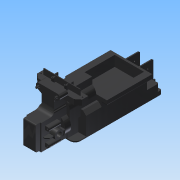
# Autodesk Inventor part: RearHousing
Saved by Autodesk Inventor 2014 (Build 180170000, 170)
## iProperties
Created: 2014-01-01
Part Number: RearHousing
Material: ABS Plastic
Document SubType Name: Modeling
Designer: davidgitz
Density: 1.06 g/cm^3
Appearance: Dark Gray
Author: davidgitz
Autodesk Inventor part; units mm, degrees
ref_plane "YZ Plane" through (0, 0, 0) normal (1, 0, 0) x (0, 1, 0)
ref_plane "XZ Plane" through (0, 0, 0) normal (0, 1, 0) x (-1, 0, 0)
ref_plane "XY Plane" through (0, 0, 0) normal (0, 0, 1) x (1, 0, 0)
sketch "Sketch1" plane through (0, 0, 0) normal (1, 0, 0) x (0, 1, 0)
  line L0 (28.5466, -43.7395) -> (-41.0494, -43.7395)
  line L1 (-41.0494, -43.7395) -> (-41.0494, 18.4905)
  line L2 (-41.0494, 18.4905) -> (-38.2554, 18.4905)
  line L3 (-38.2554, 18.4905) -> (-38.2554, 29.6665)
  line L4 (-38.2554, 29.6665) -> (20.9266, 29.6665)
  line L5 (20.9266, 29.6665) -> (20.9266, -2.0835)
  line L6 (28.5466, -43.7395) -> (28.5466, -14.2156)
  line L7 (33.9908, -15.5455) -> (15.8112, -15.5455) construction
  arc A0 (20.9266, -2.0835) -> (28.5466, -14.2156) centre (34.3947, -2.0835) ccw
  dimension "d13" = 62.23
  dimension "d15" = 2.794
  dimension "d16" = 11.176
  dimension "d17" = 59.182
  dimension "d18" = 31.75
  dimension "d19" = 28.194
  dimension "d20" = 7.62
  dimension "d21" = 69.596
  constraints: 16 end point, 5 parallel, 2 perpendicular, 2 point on circle, 1 centre point, 1 horizontal, 1 tangent
  measures "d13" distance of L0.end L1.end
  measures "d15" distance of L1.end L2.end
  measures "d16" distance of L2.end L3.end
  measures "d17" distance of L3.end L4.end
  measures "d18" distance of L4.end L5.end
  measures "d19" distance between parallel lines of L0 L7
  measures "d20" distance between parallel lines of L5 L6
  measures "d21" distance of L0.start L0.end
extrude "Extrusion1" add sketch "Sketch1" along normal mid plane 29.972
sketch "Sketch2" plane through (14.986, 0, 0) normal (1, 0, 0) x (0, 0, -1)
  line L0 (43.7395, -41.0494) -> (43.7395, 28.5466) projected
  line L1 (43.7395, 28.5466) -> (14.2156, 28.5466) projected
  arc A0 (2.0835, 20.9266) -> (14.2156, 28.5466) centre (2.0835, 34.3947) ccw projected
  line L2 (2.0835, 20.9266) -> (-29.6665, 20.9266) projected
  line L3 (-18.4905, -41.0494) -> (43.7395, -41.0494) projected
  line L4 (-18.4905, -41.0494) -> (-18.4905, 20.9266)
  point P0 (0, 0)
  constraints: 2 end point, 1 perpendicular, 1 point on line
extrude "Extrusion2" add sketch "Sketch2" along normal blind 2.54
mirror "Mirror1" about plane through (0, 0, 0) normal (1, 0, 0) of "Extrusion2"
fillet "Fillet1" radius 3.175 2 edges at (0, 20.9266, 29.6665) (0, -38.2554, 29.6665)
sketch "Sketch3" plane through (17.526, 0, 0) normal (1, 0, 0) x (0, 0, -1)
  line L0 (43.7395, -41.0494) -> (43.7395, 28.5466) projected
  line L1 (-18.4905, -41.0494) -> (43.7395, -41.0494) projected
  circle A0 centre (11.7355, -11.941) radius 10.414
  line L2 (0.9775, -22.355) -> (22.9537, -22.355) construction
  line L3 (22.1495, -2.7453) -> (22.1495, -21.5379) construction
  circle A1 centre (11.7355, -11.941) radius 6.096
  point P0 (0, 0)
  dimension "d27" = 20.828
  dimension "d28" = 18.6944
  dimension "d29" = 21.59
  dimension "d30" = 12.192
  constraints: 4 end point, 2 centre point, 2 tangent, 1 coincident, 1 parallel, 1 vertical
  measures "d27" diameter of A0
  measures "d28" distance between parallel lines of L1 L2
  measures "d29" distance between parallel lines of L0 L3
  measures "d30" diameter of A1
extrude "Extrusion3" add sketch "Sketch3" along normal blind 13.8684
sketch "Sketch4" plane through (17.526, -41.0494, -43.7395) normal (0, 0, -1) x (-1, 0, 0)
  arc A0 (0, 49.657) -> (0, 8.5598) centre (13.869, 29.1084) ccw
  line L0 (0, 49.657) -> (0, 8.5598)
  line L1 (-10.922, 46.5871) -> (-10.922, 14.6096) construction
  line L2 (0, 0) -> (35.052, 0) projected
  line L3 (0, 29.1084) -> (-28.8922, 29.1084) construction
  line L4 (0, 0) -> (0, 69.596) construction
  line L5 (0, 69.596) -> (0, 61.976) construction
  line L6 (0, 61.976) -> (0, 0) construction
  line L7 (0, 18.6944) -> (0, 39.5224) construction
  point P0 (17.526, 41.0494)
  dimension "d33" = 8.5598
  dimension "d39" = 29.1084
  dimension "d40" = 10.922
  constraints: 6 end point, 2 point on circle, 2 point on line, 1 centre point, 1 midpoint, 1 parallel, 1 perpendicular, 1 tangent
  measures "d33" distance of L2.start L0.end
  measures "d39" distance from line of L2 L3.start
  measures "d40" distance between parallel lines of L7 L1
extrude "Extrusion4" add sketch "Sketch4" against normal blind 13.97
sketch "Sketch5" plane through (17.526, 0, 0) normal (1, 0, 0) x (0, 0, -1)
  circle A0 centre (11.7355, -11.941) radius 10.414 projected
  line L0 (29.7695, -32.4896) -> (29.7695, 8.6076) projected
  line L1 (-18.4905, 20.9266) -> (-18.4905, -41.0494) projected
  line L2 (-8.7369, 10.284) -> (20.2191, 10.284)
  line L3 (20.2191, 10.284) -> (20.2191, 1.267)
  line L4 (20.2191, 1.267) -> (-8.7369, 1.267)
  line L5 (-8.7369, 1.267) -> (-8.7369, 10.284)
  line L6 (-8.2035, -11.941) -> (34.9388, -11.941) construction
  line L7 (-13.9185, -11.941) -> (-13.9185, -10.925)
  line L8 (-13.9185, -10.925) -> (1.3712, -10.925)
  line L9 (22.0998, -10.925) -> (29.7695, -10.925)
  line L10 (-5.7611, -1.527) -> (23.7536, -1.527) construction
  line L11 (-8.7369, -34.166) -> (20.2191, -34.166)
  line L12 (20.2191, -34.166) -> (20.2191, -25.149)
  line L13 (20.2191, -25.149) -> (-8.7369, -25.149)
  line L14 (-8.7369, -25.149) -> (-8.7369, -34.166)
  line L15 (-13.9185, -11.941) -> (-13.9185, -12.957)
  line L16 (-13.9185, -12.957) -> (1.3712, -12.957)
  line L17 (22.0998, -12.957) -> (29.7695, -12.957)
  arc A1 (1.3712, -10.925) -> (1.3712, -12.957) centre (11.7355, -11.941) ccw
  arc A2 (22.0998, -12.957) -> (22.0998, -10.925) centre (11.7355, -11.941) ccw
  line L18 (29.7695, -10.925) -> (29.7695, -12.957)
  point P0 (0, 0)
  point P1 (29.7695, -11.941)
  dimension "d41" = 28.956
  dimension "d42" = 9.017
  dimension "d43" = 9.7536
  dimension "d44" = 2.794
  dimension "d45" = 2.032
  dimension "d46" = 15.24
  constraints: 34 end point, 8 symmetric about line, 6 point on circle, 5 perpendicular, 4 point on line, 3 parallel, 2 centre point, 2 collinear, 1 coincident, 1 horizontal, 1 midpoint, 1 tangent
  measures "d41" distance of L2.start L2.end
  measures "d42" distance between parallel lines of L4 L2
  measures "d43" distance between parallel lines of L5 L1
  measures "d44" distance between parallel lines of L10 L4
  measures "d45" distance between parallel lines of L8 L16
  measures "d46" distance edge to line of A0 L7
extrude "Extrusion5" add sketch "Sketch5" along normal blind 10.16 contours A0 L9 L0 L17 | A0 L16 L15 L7 L8 | L2 L3 L4 L5 | L14 L13 L12 L11
chamfer "Chamfer1" distance 6.35 angle 45 1 edges at (27.686, -11.941, 13.9185)
sketch "Sketch6" plane through (17.526, 1.267, 8.7369) normal (0, 0, 1) x (1, 0, 0)
  line L0 (0, 0) -> (10.16, 0) projected
  circle A0 centre (5.6515, 4.5085) radius 1.5875
  arc A1 (10.16, 4.5085) -> (5.6515, 9.017) centre (5.6515, 4.5085) ccw
  line L1 (5.6515, 9.017) -> (10.16, 9.017)
  line L2 (10.16, 9.017) -> (10.16, 4.5085)
  line L3 (5.6515, 4.5085) -> (8.0267, 4.5085) construction
  arc A2 (5.6515, 0) -> (10.16, 4.5085) centre (5.6515, 4.5085) ccw
  line L4 (5.6515, 0) -> (10.16, 0)
  line L5 (10.16, 0) -> (10.16, 4.5085)
  point P0 (-17.526, -1.267)
  dimension "d52" = 3.175
  constraints: 10 end point, 4 point on circle, 3 centre point, 3 symmetric about line, 2 point on line, 1 coincident, 1 perpendicular, 1 tangent, 1 other
  measures "d52" diameter of A0
extrude "Extrusion6" cut sketch "Sketch6" against normal up to next
ref_plane "Work Plane1" through (17.526, -11.941, -11.7355) normal (0, 1, 0) x (1, 0, 0)
mirror "Mirror2" about plane through (17.526, -11.941, -11.7355) normal (0, 1, 0) of "Extrusion6"
mirror "Mirror3" about plane through (0, 0, 0) normal (1, 0, 0) of "Extrusion3", "Extrusion4", "Extrusion5", "Chamfer1", "Extrusion6", "Mirror2"
sketch "Sketch7" plane through (0, 0, 0) normal (1, 0, 0) x (0, 1, 0)
  arc A0 (28.5466, -14.2156) -> (34.3947, -15.5515) centre (34.3947, -2.0835) ccw
  arc A1 (20.9266, -2.0835) -> (28.5466, -14.2156) centre (34.3947, -2.0835) ccw projected
  line L0 (28.5466, -43.7395) -> (28.5466, -14.2156) projected
  line L1 (8.6076, -43.7395) -> (28.5466, -43.7395) projected
  line L2 (28.5466, -14.2156) -> (28.5466, -43.7395)
  line L3 (28.5466, -43.7395) -> (38.1986, -43.7395)
  line L4 (38.1986, -43.7395) -> (38.1986, -108.7635)
  line L5 (38.1986, -108.7635) -> (54.4546, -108.7635)
  line L6 (54.4546, -108.7635) -> (54.4546, -58.9795)
  line L7 (54.4546, -58.9795) -> (58.2646, -58.9795)
  line L8 (58.2646, -58.9795) -> (58.2646, -15.5515)
  line L9 (58.2646, -15.5515) -> (34.3947, -15.5515)
  line L10 (54.1292, -15.5515) -> (12.3088, -15.5515) construction
  point P0 (0, 0)
  dimension "d57" = 9.652
  dimension "d58" = 65.024
  dimension "d59" = 16.256
  dimension "d60" = 49.784
  dimension "d61" = 3.81
  dimension "d62" = 43.4279
  dimension "d63" = 29.718
  constraints: 18 end point, 5 parallel, 3 collinear, 2 concentric, 2 perpendicular, 2 point on circle, 1 centre point, 1 point on line, 1 tangent
  measures "d57" distance of L0.start L3.end
  measures "d58" distance of L3.end L4.end
  measures "d59" distance of L4.end L5.end
  measures "d60" distance of L5.end L6.end
  measures "d61" distance of L6.end L7.end
  measures "d62" distance of L7.end L8.end
  measures "d63" distance between parallel lines of L2 L8
extrude "Extrusion7" add sketch "Sketch7" along normal mid plane 29.972
fillet "Fillet2" radius 3.175 2 edges at (17.526, 28.5466, -28.9775) (-17.526, 28.5466, -28.9775)
fillet "Fillet3" radius 3.175 2 edges at (-14.986, 28.5466, -28.9775) (14.986, 28.5466, -28.9775)
sketch "Sketch9" plane through (-14.986, 34.3947, -15.5515) normal (0, 0, 1) x (1, 0, 0)
  line L0 (29.972, 23.8699) -> (29.972, 0) projected
  line L1 (0, 23.8699) -> (29.972, 23.8699) projected
  line L2 (0, 23.8699) -> (29.972, 23.8699)
  line L3 (29.972, 23.8699) -> (29.972, 11.4239)
  line L4 (29.972, 11.4239) -> (0, 11.4239)
  line L5 (0, 11.4239) -> (0, 23.8699)
  point P0 (14.986, -34.3947)
  dimension "d69" = 12.446
  constraints: 8 end point, 2 parallel, 1 horizontal, 1 perpendicular, 1 point on line
  measures "d69" distance between parallel lines of L1 L4
extrude "Extrusion8" cut sketch "Sketch9" against normal blind 19.558
sketch "Sketch10" plane through (-14.986, 34.3947, -35.1095) normal (0, 0, 1) x (1, 0, 0)
  line L0 (29.972, 23.8699) -> (29.972, 11.4239) projected
  line L1 (29.972, 11.4239) -> (0, 11.4239) projected
  line L2 (29.972, 11.4239) -> (29.972, 13.8369)
  line L3 (31.6529, 16.6384) -> (40.8193, 21.5272)
  line L4 (42.7792, 32.0645) -> (41.5897, 33.4399)
  line L5 (39.1882, 34.5379) -> (14.986, 34.5379)
  line L6 (14.986, 34.5379) -> (14.986, 11.4239) construction
  arc A0 (40.8193, 21.5272) -> (42.7792, 32.0645) centre (37.592, 27.5783) ccw
  line L7 (44.45, 35.5945) -> (44.45, 20.8192) construction
  arc A1 (41.5897, 33.4399) -> (39.1882, 34.5379) centre (39.1882, 31.3629) ccw
  arc A2 (31.6529, 16.6384) -> (29.972, 13.8369) centre (33.147, 13.8369) ccw
  line L8 (0, 13.8369) -> (0, 11.4239)
  line L9 (0, 11.4239) -> (0, 13.8369)
  line L10 (-1.6809, 16.6384) -> (-10.8473, 21.5272)
  line L11 (-12.8072, 32.0645) -> (-11.6177, 33.4399)
  line L12 (-9.2162, 34.5379) -> (14.986, 34.5379)
  arc A3 (-12.8072, 32.0645) -> (-10.8473, 21.5272) centre (-7.62, 27.5783) ccw
  line L13 (-14.478, 35.5945) -> (-14.478, 20.8192) construction
  arc A4 (-9.2162, 34.5379) -> (-11.6177, 33.4399) centre (-9.2162, 31.3629) ccw
  arc A5 (0, 13.8369) -> (-1.6809, 16.6384) centre (-3.175, 13.8369) ccw
  line L14 (29.972, 11.4239) -> (0, 11.4239)
  point P0 (14.986, -34.3947)
  point P1 (29.972, 15.7419)
  point P2 (40.64, 34.5379)
  point P3 (0, 15.7419)
  point P4 (-10.668, 34.5379)
  dimension "d72" = 23.114
  dimension "d73" = 6.9596
  dimension "d74" = 7.62
  dimension "d75" = 4.318
  dimension "d76" = 14.478
  dimension "d77" = 10.668
  dimension "d78" = 3.175
  constraints: 26 end point, 13 symmetric about line, 12 point on circle, 10 point on line, 7 tangent, 6 centre point, 1 collinear, 1 equal radius, 1 midpoint, 1 parallel, 1 perpendicular, 3 other
  measures "d72" distance between parallel lines of L1 L5
  measures "d73" distance from line of A0.centre L5
  measures "d74" distance from line of L0 A0.centre
  measures "d75" distance from line of L1 point (29.972, 15.742)
  measures "d76" distance between parallel lines of L0 L7
  measures "d77" distance from line of point (40.64, 34.538) L0
  measures "d78" radius of A1
extrude "Extrusion9" add sketch "Sketch10" along normal blind 19.558
sketch "Sketch11" plane through (-14.986, 34.3947, -15.5515) normal (0, 0, 1) x (1, 0, 0)
  line L0 (0, 0) -> (29.972, 0) projected
  arc A0 (40.8193, 21.5272) -> (42.7792, 32.0645) centre (37.592, 27.5783) ccw projected
  line L1 (39.1882, 34.5379) -> (-9.2162, 34.5379) projected
  line L2 (14.986, 0) -> (14.986, 35.0273) construction
  circle A1 centre (37.592, 27.5783) radius 2.54
  circle A2 centre (37.592, 27.5783) radius 1.27
  circle A3 centre (-7.62, 27.5783) radius 2.54
  circle A4 centre (-7.62, 27.5783) radius 1.27
  point P0 (14.986, -34.3947)
  dimension "d81" = 5.08
  dimension "d83" = 2.54
  dimension "d84" = 40.132
  constraints: 4 centre point, 3 coincident, 2 end point, 2 symmetric about line, 1 midpoint, 1 perpendicular, 2 other
  measures "d81" diameter of A1
  measures "d83" diameter of A2
extrude "Extrusion10" add sketch "Sketch11" along normal blind 6.096
sketch "Sketch12" plane through (-14.986, 58.2646, -58.9795) normal (0, 1, 0) x (1, 0, 0)
  line L0 (0, -23.8699) -> (29.972, -23.8699) projected
  line L1 (29.972, 0) -> (29.972, -23.8699) projected
  line L2 (0, 0) -> (29.972, 0) projected
  line L3 (0, -23.8699) -> (0, 0) projected
  line L4 (14.986, -23.8699) -> (14.986, 0) construction
  line L5 (14.986, 0) -> (70.104, 0)
  line L6 (70.104, 0) -> (70.104, -14.8844)
  line L7 (70.104, -14.8844) -> (59.182, -23.8699)
  line L8 (59.182, -23.8699) -> (14.986, -23.8699)
  circle A0 centre (65.532, -9.398) radius 1.5875
  line L9 (14.986, 0) -> (-40.132, 0)
  line L10 (-40.132, 0) -> (-40.132, -14.8844)
  line L11 (-40.132, -14.8844) -> (-29.21, -23.8699)
  line L12 (-29.21, -23.8699) -> (14.986, -23.8699)
  circle A1 centre (-35.56, -9.398) radius 1.5875
  point P0 (14.986, -58.9795)
  dimension "d87" = 29.21
  dimension "d88" = 40.132
  dimension "d89" = 3.175
  dimension "d90" = 9.398
  dimension "d91" = 4.572
  dimension "d92" = 14.8844
  constraints: 18 end point, 4 symmetric about line, 2 centre point, 2 midpoint, 1 parallel, 1 perpendicular, 1 vertical, 1 other
  measures "d87" distance from line of L7.end L1
  measures "d88" distance between parallel lines of L1 L6
  measures "d89" diameter of A0
  measures "d90" distance from line of L5 A0.centre
  measures "d91" distance from line of L6 A0.centre
  measures "d92" distance of L5.end L6.end
extrude "Extrusion11" add sketch "Sketch12" against normal blind 12.954 contours L12 L11 L10 L9 L3 | L1 L5 L6 L7 L8
sketch "Sketch13" plane through (-14.986, 45.3106, -58.9795) normal (0, -1, 0) x (1, 0, 0)
  line L0 (29.972, 0) -> (29.972, 23.8699) projected
  line L1 (29.972, 0) -> (70.104, 0) projected
  line L2 (70.104, 0) -> (70.104, 14.8844) projected
  line L3 (70.104, 14.8844) -> (59.182, 23.8699) projected
  line L4 (59.182, 23.8699) -> (29.972, 23.8699) projected
  circle A0 centre (65.532, 9.398) radius 1.5875 projected
  line L5 (32.004, 21.8379) -> (32.004, 2.032)
  line L6 (32.004, 2.032) -> (68.072, 2.032)
  line L7 (68.072, 2.032) -> (68.072, 13.9248)
  line L8 (68.072, 13.9248) -> (58.4536, 21.8379)
  line L9 (58.4536, 21.8379) -> (32.004, 21.8379)
  circle A1 centre (65.532, 9.398) radius 1.5875
  point P0 (14.986, 58.9795)
  dimension "d95" = 2.032
  constraints: 10 end point, 1 centre point, 1 coincident, 1 concentric, 4 other
  measures "d95" distance between parallel lines of L4 L9
extrude "Extrusion12" cut sketch "Sketch13" against normal blind 11.938 contours L9 L8 L7 L6 L5
mirror "Mirror4" about plane through (0, 0, 0) normal (1, 0, 0) of "Extrusion12"
sketch "Sketch14" plane through (17.526, -41.0494, -43.7395) normal (0, 0, -1) x (-1, 0, 0)
  line L0 (32.512, 79.248) -> (2.54, 79.248) projected
  arc A0 (1.27, 69.0251) -> (2.54, 71.5651) centre (-0.635, 71.5651) ccw projected
  arc A1 (1.27, 69.0251) -> (0, 66.4851) centre (3.175, 66.4851) ccw projected
  line L1 (0, 49.657) -> (0, 66.4851) projected
  line L2 (0, 0) -> (35.052, 0) projected
  line L3 (35.052, 49.657) -> (35.052, 66.4851) projected
  line L4 (-7.62, 35.56) -> (-7.62, 60.96)
  line L5 (2.54, 89.281) -> (2.54, 75.4441) projected
  arc A2 (2.54, 79.248) -> (-7.62, 60.96) centre (13.9192, 60.96) ccw
  line L6 (-26.67, 86.36) -> (2.54, 86.36) projected
  line L7 (-7.62, 35.56) -> (17.526, 35.56)
  line L8 (17.526, 79.248) -> (17.526, 0) construction
  line L9 (2.54, 79.248) -> (17.526, 79.248)
  line L10 (32.512, 71.5651) -> (32.512, 79.248)
  arc A3 (32.512, 71.5651) -> (33.782, 69.0251) centre (35.687, 71.5651) ccw
  arc A4 (35.052, 66.4851) -> (33.782, 69.0251) centre (31.877, 66.4851) ccw
  line L11 (35.052, 49.657) -> (35.052, 66.4851)
  line L12 (42.672, 35.56) -> (42.672, 60.96)
  arc A5 (42.672, 60.96) -> (32.512, 79.248) centre (21.1328, 60.96) ccw
  line L13 (42.672, 35.56) -> (17.526, 35.56)
  line L14 (32.512, 79.248) -> (17.526, 79.248)
  point P0 (17.526, 41.0494)
  point P1 (32.512, 75.4441)
  dimension "d100" = 7.62
  dimension "d101" = 25.4
  dimension "d103" = 35.56
  constraints: 18 end point, 8 point on circle, 6 symmetric about line, 4 centre point, 2 midpoint, 2 parallel, 1 collinear, 1 point on line, 1 tangent, 3 other
  measures "d100" distance between parallel lines of L1 L4
  measures "d101" distance of L4.start L4.end
  measures "d103" distance between parallel lines of L7 L2
extrude "Extrusion13" add sketch "Sketch14" along normal up to surface (65.024 mm away)
sketch "Sketch15" plane through (28.3749, 58.2646, -35.1095) normal (0, 1, 0) x (1, 0, 0)
  line L0 (0, 0) -> (-56.7498, 0) projected
  line L1 (-83.4929, 23.8699) -> (26.7431, 23.8699) projected
  line L2 (-72.5709, 0) -> (-56.7498, 0) projected
  line L3 (-73.2059, 15.9959) -> (-73.2059, 14.2179)
  line L4 (16.4561, 14.2179) -> (16.4561, 15.9959)
  line L5 (-73.2059, 14.2179) -> (-28.3749, 14.2179)
  line L6 (-23.6446, 14.2179) -> (6.4493, 14.2179)
  line L7 (-28.3749, 14.2179) -> (16.4561, 14.2179)
  line L8 (-28.3749, 23.8699) -> (-28.3749, 0) construction
  line L9 (-83.4929, 23.8699) -> (-83.4929, 8.9855) projected
  line L10 (-48.125, 15.9959) -> (-48.125, 23.8699)
  line L11 (-48.125, 23.8699) -> (-46.347, 23.8699)
  line L12 (-46.347, 23.8699) -> (-46.347, 15.9959)
  line L13 (-10.4028, 15.9959) -> (-10.4028, 23.8699)
  line L14 (-10.4028, 23.8699) -> (-8.6248, 23.8699)
  line L15 (-8.6248, 23.8699) -> (-8.6248, 15.9959)
  line L16 (-46.347, 23.8699) -> (-10.4028, 23.8699) construction
  line L17 (-48.125, 15.9959) -> (-73.2059, 15.9959)
  line L18 (16.4561, 15.9959) -> (-8.6248, 15.9959)
  line L19 (-10.4028, 15.9959) -> (-46.347, 15.9959)
  point P0 (-28.3749, -35.1095)
  point P1 (-28.3749, 15.9959)
  point P2 (-28.3749, 23.8699)
  dimension "d112" = 89.662
  dimension "d114" = 7.874
  dimension "d115" = 1.778
  constraints: 32 end point, 11 parallel, 10 perpendicular, 5 point on line, 4 collinear, 4 midpoint, 3 equal length, 3 horizontal, 1 vertical
  measures "d112" distance between parallel lines of L4 L3
  measures "d114" distance between parallel lines of L19 L1
  measures "d115" distance of L4.start L4.end
extrude "Extrusion14" add sketch "Sketch15" along normal blind 13.6652 contours L1 L12 L19 L13 L15 L18 L4 L7 L6 L5 L3 L17 L10
sketch "Sketch16" plane through (-44.196, 58.2646, -35.1095) normal (0, 1, 0) x (1, 0, 0)
  line L0 (89.027, 14.2179) -> (-0.635, 14.2179) projected
  line L1 (72.5709, 0) -> (15.8211, 0) projected
  line L2 (44.196, 14.2179) -> (44.196, 6.9151) construction
  arc A0 (59.182, 10.9921) -> (60.96, 10.9921) centre (60.071, 8.2097) ccw
  circle A1 centre (60.071, 8.2097) radius 1.27
  line L3 (59.182, 14.2179) -> (59.182, 10.9921)
  line L4 (59.182, 14.2179) -> (60.96, 14.2179)
  line L5 (60.96, 10.9921) -> (60.96, 14.2179)
  arc A2 (27.432, 10.9921) -> (29.21, 10.9921) centre (28.321, 8.2097) ccw
  circle A3 centre (28.321, 8.2097) radius 1.27
  line L6 (29.21, 14.2179) -> (29.21, 10.9921)
  line L7 (29.21, 14.2179) -> (27.432, 14.2179)
  line L8 (27.432, 10.9921) -> (27.432, 14.2179)
  point P0 (44.196, -35.1095)
  dimension "d116" = 1.778
  dimension "d118" = 5.842
  dimension "d119" = 2.54
  dimension "d120" = 29.972
  dimension "d121" = 3.2258
  constraints: 14 end point, 6 symmetric about line, 4 centre point, 4 point on circle, 2 coincident, 2 parallel, 2 perpendicular, 2 point on line, 1 midpoint, 2 other
  measures "d116" distance of L3.start L4.end
  measures "d118" diameter of A0
  measures "d119" diameter of A1
  measures "d120" distance between parallel lines of L3 L6
  measures "d121" distance of L5.start L4.end
extrude "Extrusion15" add sketch "Sketch16" along normal blind 11.938
sketch "Sketch17" plane through (14.986, 54.4546, -108.7635) normal (0, 0, -1) x (-1, 0, 0)
  line L0 (-10.16, -59.944) -> (-10.16, -34.544) projected
  line L1 (40.132, -59.944) -> (-10.16, -59.944) projected
  line L2 (40.132, -34.544) -> (40.132, -59.944) projected
  line L3 (45.212, -44.4812) -> (53.34, -52.6092)
  line L4 (53.34, -52.6092) -> (53.34, -98.806)
  line L5 (53.34, -98.806) -> (14.986, -98.806)
  line L6 (45.212, -44.4812) -> (40.132, -44.4812)
  line L7 (14.986, -44.4812) -> (14.986, -98.806) construction
  line L8 (-2.54, -95.504) -> (32.512, -95.504) construction
  line L9 (-15.24, -44.4812) -> (-23.368, -52.6092)
  line L10 (-23.368, -52.6092) -> (-23.368, -98.806)
  line L11 (-23.368, -98.806) -> (14.986, -98.806)
  line L12 (-15.24, -44.4812) -> (-10.16, -44.4812)
  line L13 (-10.16, -44.4812) -> (-10.16, -59.944)
  line L14 (-10.16, -59.944) -> (40.132, -59.944)
  line L15 (40.132, -59.944) -> (40.132, -44.4812)
  point P0 (14.986, -54.4546)
  dimension "d124" = 5.08
  dimension "d125" = 45
  dimension "d126" = 13.208
  dimension "d127" = 3.302
  constraints: 24 end point, 4 perpendicular, 3 point on line, 3 symmetric about line, 1 collinear, 1 parallel
  measures "d124" distance from line of L3.start L2
  measures "d125" angle of L3 L6
  measures "d126" distance between parallel lines of L2 L4
  measures "d127" distance between parallel lines of L8 L5
extrude "Extrusion16" add sketch "Sketch17" against normal blind 38.1
sketch "Sketch18" plane through (14.986, 54.4546, -70.6635) normal (0, 0, 1) x (1, 0, 0)
  line L0 (-40.132, -59.944) -> (10.16, -59.944) projected
  line L1 (-53.34, -98.806) -> (23.368, -98.806) projected
  line L2 (23.368, -98.806) -> (23.368, -52.6092) projected
  line L3 (-14.986, -59.944) -> (4.318, -59.944)
  line L4 (4.318, -59.944) -> (4.318, -96.266)
  line L5 (4.318, -96.266) -> (23.368, -96.266)
  line L6 (23.368, -98.806) -> (23.368, -96.266)
  line L7 (23.368, -98.806) -> (-14.986, -98.806)
  line L8 (-14.986, -59.944) -> (-14.986, -98.806) construction
  line L9 (-53.34, -98.806) -> (-53.34, -96.266)
  line L10 (-14.986, -59.944) -> (-34.29, -59.944)
  line L11 (-34.29, -59.944) -> (-34.29, -96.266)
  line L12 (-34.29, -96.266) -> (-53.34, -96.266)
  line L13 (-53.34, -98.806) -> (-53.34, -96.266)
  line L14 (-53.34, -98.806) -> (-14.986, -98.806)
  point P0 (-14.986, -54.4546)
  dimension "d131" = 2.54
  dimension "d134" = 19.05
  constraints: 24 end point, 3 perpendicular, 3 symmetric about line, 2 midpoint, 2 point on line, 1 collinear
  measures "d131" distance between parallel lines of L1 L5
  measures "d134" distance between parallel lines of L2 L4
extrude "Extrusion17" add sketch "Sketch18" along normal up to surface (26.924 mm away)
sketch "Sketch19" plane through (14.986, 54.4546, -108.7635) normal (0, 0, -1) x (-1, 0, 0)
  arc A0 (0, -16.256) -> (-10.16, -34.544) centre (11.3792, -34.544) ccw projected
  arc A1 (40.132, -34.544) -> (29.972, -16.256) centre (18.5928, -34.544) ccw projected
  line L0 (-23.368, -98.806) -> (53.34, -98.806) projected
  line L1 (14.986, -98.806) -> (53.34, -98.806)
  line L2 (53.34, -98.806) -> (53.34, -44.196)
  line L3 (53.34, -44.196) -> (66.04, -44.196)
  line L4 (66.04, -44.196) -> (66.04, -32.258)
  line L5 (66.04, -32.258) -> (14.986, -32.258)
  line L6 (14.986, -98.806) -> (14.986, -32.258) construction
  line L7 (14.986, -98.806) -> (-23.368, -98.806)
  line L8 (-23.368, -98.806) -> (-23.368, -44.196)
  line L9 (-23.368, -44.196) -> (-36.068, -44.196)
  line L10 (-36.068, -44.196) -> (-36.068, -32.258)
  line L11 (-36.068, -32.258) -> (14.986, -32.258)
  point P0 (18.5928, -34.544)
  point P1 (11.3792, -34.544)
  dimension "d136" = 54.61
  dimension "d137" = 12.7
  dimension "d138" = 11.938
  constraints: 22 end point, 5 symmetric about line, 3 perpendicular, 2 parallel, 1 collinear, 1 midpoint
  measures "d136" distance of L0.end L2.end
  measures "d137" distance of L2.end L3.end
  measures "d138" distance of L3.end L4.end
extrude "Extrusion18" add sketch "Sketch19" along normal blind 110.998
sketch "Sketch20" plane through (-38.354, -44.3514, -43.7395) normal (0, -1, 0) x (1, 0, 0)
  line L0 (76.708, -176.022) -> (0, -176.022) projected
  line L1 (0, -176.022) -> (76.708, -176.022)
  line L2 (76.708, -176.022) -> (76.708, -211.582)
  line L3 (76.708, -211.582) -> (0, -211.582)
  line L4 (0, -211.582) -> (0, -176.022)
  point P0 (38.354, 43.7395)
  dimension "d144" = 35.56
  constraints: 8 end point, 2 parallel, 1 horizontal, 1 perpendicular
  measures "d144" distance of L0.start L2.end
extrude "Extrusion19" add sketch "Sketch20" against normal blind 9.525
sketch "Sketch21" plane through (-38.354, -34.8264, -43.7395) normal (0, 1, 0) x (1, 0, 0)
  line L0 (76.708, 176.022) -> (0, 176.022) projected
  line L1 (76.708, 176.022) -> (76.708, 211.582) projected
  line L2 (0, 176.022) -> (76.708, 176.022)
  line L3 (76.708, 176.022) -> (76.708, 204.6986)
  line L4 (76.708, 204.6986) -> (0, 204.6986)
  line L5 (0, 204.6986) -> (0, 176.022)
  point P0 (38.354, -43.7395)
  dimension "d143" = 28.6766
  constraints: 8 end point, 2 parallel, 1 horizontal, 1 perpendicular, 1 point on line
  measures "d143" distance between parallel lines of L0 L4
extrude "Extrusion20" add sketch "Sketch21" along normal blind 17.018
sketch "Sketch22" plane through (-38.354, -17.8084, -43.7395) normal (0, 1, 0) x (1, 0, 0)
  line L0 (76.708, 204.6986) -> (0, 204.6986) projected
  line L1 (38.354, 204.6986) -> (38.354, 176.022) construction
  line L2 (23.241, 176.022) -> (23.241, 212.09)
  line L3 (23.241, 212.09) -> (20.701, 212.09)
  line L4 (20.701, 212.09) -> (20.701, 176.022)
  line L5 (53.467, 176.022) -> (53.467, 212.09)
  line L6 (53.467, 212.09) -> (56.007, 212.09)
  line L7 (56.007, 212.09) -> (56.007, 176.022)
  line L8 (20.701, 176.022) -> (23.241, 176.022)
  line L9 (53.467, 176.022) -> (56.007, 176.022)
  point P0 (38.354, -43.7395)
  dimension "d147" = 2.54
  dimension "d148" = 36.068
  dimension "d149" = 30.226
  constraints: 18 end point, 4 symmetric about line, 2 perpendicular, 1 collinear, 1 midpoint, 1 parallel
  measures "d147" distance of L2.end L3.end
  measures "d148" distance of L2.start L2.end
  measures "d149" distance between parallel lines of L2 L5
extrude "Extrusion21" add sketch "Sketch22" along normal blind 37.338
sketch "Sketch23" plane through (-38.354, -17.8084, -43.7395) normal (0, -1, 0) x (1, 0, 0)
  line L0 (53.467, -212.09) -> (56.007, -212.09)
  line L1 (56.007, -212.09) -> (56.007, -204.6986)
  line L2 (56.007, -204.6986) -> (53.467, -204.6986)
  line L3 (53.467, -204.6986) -> (53.467, -212.09)
  line L4 (20.701, -176.022) -> (0, -176.022) projected
  line L5 (0, -176.022) -> (-12.7, -176.022) projected
  line L6 (-12.7, -176.022) -> (89.408, -176.022) projected
  line L7 (89.408, -176.022) -> (76.708, -176.022) projected
  line L8 (76.708, -176.022) -> (56.007, -176.022) projected
  line L9 (56.007, -176.022) -> (53.467, -176.022) projected
  line L10 (53.467, -176.022) -> (23.241, -176.022) projected
  line L11 (23.241, -176.022) -> (20.701, -176.022) projected
  line L12 (38.354, -176.022) -> (38.354, -242.3481) construction
  line L13 (20.701, -204.6986) -> (23.241, -204.6986)
  line L14 (23.241, -204.6986) -> (23.241, -212.09)
  line L15 (23.241, -212.09) -> (20.701, -212.09)
  line L16 (20.701, -212.09) -> (20.701, -204.6986)
  line L17 (23.241, -212.09) -> (20.701, -212.09)
  line L18 (20.701, -212.09) -> (20.701, -204.6986)
  line L19 (20.701, -204.6986) -> (23.241, -204.6986)
  line L20 (23.241, -204.6986) -> (23.241, -212.09)
  point P0 (38.354, 43.7395)
  constraints: 26 end point, 6 symmetric about line, 2 parallel, 2 perpendicular, 1 horizontal, 1 midpoint
extrude "Extrusion22" add sketch "Sketch23" along normal up to surface (17.018 mm away)
sketch "Sketch24" plane through (-38.354, -44.3514, -43.7395) normal (0, -1, 0) x (1, 0, 0)
  line L0 (0, -211.582) -> (76.708, -211.582) projected
  line L1 (20.701, -222.758) -> (56.007, -222.758)
  line L2 (56.007, -222.758) -> (56.007, -211.582)
  line L3 (56.007, -211.582) -> (20.701, -211.582)
  line L4 (20.701, -211.582) -> (20.701, -222.758)
  line L5 (20.701, -176.022) -> (20.701, -204.6986) projected
  line L6 (20.701, -212.09) -> (20.701, -176.022) projected
  line L7 (20.701, -212.09) -> (20.701, -211.582) projected
  line L8 (20.701, -204.6986) -> (20.701, -211.582) projected
  line L9 (56.007, -176.022) -> (56.007, -212.09) projected
  line L10 (56.007, -204.6986) -> (56.007, -176.022) projected
  line L11 (56.007, -211.582) -> (56.007, -204.6986) projected
  line L12 (56.007, -211.582) -> (56.007, -212.09) projected
  point P0 (38.354, 43.7395)
  point P1 (38.354, -211.582)
  dimension "d154" = 11.176
  constraints: 8 end point, 2 midpoint, 2 parallel, 1 horizontal, 1 perpendicular, 1 point on line
  measures "d154" distance between parallel lines of L1 L0
extrude "Extrusion23" add sketch "Sketch24" against normal blind 3.429
sketch "Sketch25" plane through (-38.354, -40.9224, -43.7395) normal (0, 1, 0) x (1, 0, 0)
  line L0 (56.007, 211.582) -> (20.701, 211.582) projected
  line L1 (56.007, 211.582) -> (56.007, 222.758) projected
  line L2 (20.701, 176.022) -> (20.701, 204.6986) projected
  line L3 (20.701, 212.09) -> (20.701, 176.022) projected
  line L4 (20.701, 212.09) -> (20.701, 211.582) projected
  line L5 (20.701, 204.6986) -> (20.701, 211.582) projected
  line L6 (23.241, 204.6986) -> (23.241, 176.022) projected
  line L7 (23.241, 211.582) -> (23.241, 204.6986) projected
  line L8 (23.241, 211.582) -> (23.241, 212.09) projected
  line L9 (23.241, 176.022) -> (23.241, 212.09) projected
  line L10 (53.467, 176.022) -> (53.467, 204.6986) projected
  line L11 (53.467, 212.09) -> (53.467, 176.022) projected
  line L12 (53.467, 212.09) -> (53.467, 211.582) projected
  line L13 (53.467, 204.6986) -> (53.467, 211.582) projected
  line L14 (56.007, 176.022) -> (56.007, 212.09) projected
  line L15 (56.007, 204.6986) -> (56.007, 176.022) projected
  line L16 (56.007, 211.582) -> (56.007, 204.6986) projected
  line L17 (56.007, 211.582) -> (56.007, 212.09) projected
  line L18 (20.701, 211.582) -> (23.241, 211.582)
  line L19 (23.241, 211.582) -> (23.241, 216.916)
  line L20 (23.241, 216.916) -> (20.701, 216.916)
  line L21 (20.701, 216.916) -> (20.701, 211.582)
  line L22 (53.467, 211.582) -> (56.007, 211.582)
  line L23 (56.007, 211.582) -> (56.007, 216.916)
  line L24 (56.007, 216.916) -> (53.467, 216.916)
  line L25 (53.467, 216.916) -> (53.467, 211.582)
  point P0 (38.354, -43.7395)
  dimension "d157" = 5.334
  constraints: 16 end point, 4 parallel, 2 horizontal, 2 perpendicular, 1 collinear, 1 point on line
  measures "d157" distance between parallel lines of L0 L20
extrude "Extrusion24" add sketch "Sketch25" along normal blind 15.24
sketch "Sketch26" plane through (15.113, -34.8264, -255.3215) normal (0, 0, -1) x (-1, 0, 0)
  line L0 (0, 17.018) -> (30.226, 17.018) projected
  line L1 (30.226, 17.018) -> (0, 17.018)
  line L2 (0, 17.018) -> (0, -6.096)
  line L3 (0, -6.096) -> (30.226, -6.096)
  line L4 (30.226, -6.096) -> (30.226, 17.018)
  point P0 (15.113, 34.8264)
  constraints: 8 end point, 2 parallel, 1 horizontal, 1 perpendicular
extrude "Extrusion25" cut sketch "Sketch26" against normal up to surface (6.8834 mm away)
fillet "Fillet4" radius 12.7 2 edges at (38.354, -43.0814, -43.7395) (-38.354, -43.0814, -43.7395)
fillet "Fillet5" radius 3.175 12 edges at (16.383, 19.5296, -255.8295) (-16.383, 19.5296, -255.8295) (38.354, -39.5889, -255.3215) (-38.354, -39.5889, -255.3215) (38.354, -26.3174, -248.4381) (-38.354, -26.3174, -248.4381) (44.704, 10.2586, -219.7615) (51.054, 10.2586, -164.2625) (44.704, 10.2586, -108.7635) (-44.704, 10.2586, -219.7615) (-51.054, 10.2586, -164.2625) (-44.704, 10.2586, -108.7635)
sketch "Sketch27" plane through (17.653, -17.8084, -219.7615) normal (1, 0, 0) x (0, 0, -1)
  line L0 (0, 37.338) -> (32.893, 37.338) projected
  line L1 (0, 0) -> (0, 37.338) projected
  line L2 (28.6766, -17.018) -> (28.6766, 0) projected
  circle A0 centre (22.606, 23.114) radius 1.5875
  circle A1 centre (32.9946, -12.954) radius 1.5875
  circle A2 centre (3.81, 33.0962) radius 1.5875
  point P0 (-219.7615, 17.8084)
  dimension "d164" = 3.175
  dimension "d165" = 4.2418
  dimension "d166" = 14.224
  dimension "d167" = 50.292
  dimension "d168" = 3.81
  dimension "d169" = 22.606
  dimension "d171" = 4.318
  constraints: 3 centre point, 2 equal radius
  measures "d164" diameter of A0
  measures "d165" distance from line of L0 A2.centre
  measures "d166" distance from line of L0 A0.centre
  measures "d167" distance from line of A1.centre L0
  measures "d168" distance from line of L1 A2.centre
  measures "d169" distance from line of L1 A0.centre
  measures "d171" distance from line of L2 A1.centre
extrude "Extrusion26" cut sketch "Sketch27" against normal through all
sketch "Sketch28" plane through (-17.653, -44.3514, -266.4975) normal (0, -1, 0) x (1, 0, 0)
  line L0 (56.007, 210.058) -> (56.007, 14.351) projected
  line L1 (-20.701, 210.058) -> (-20.701, 14.351) projected
  line L2 (-20.701, 112.2045) -> (56.007, 112.2045) construction
  line L3 (-7.112, 184.3405) -> (42.418, 184.3405)
  line L4 (42.418, 184.3405) -> (42.418, 40.0685)
  line L5 (42.418, 40.0685) -> (-7.112, 40.0685)
  line L6 (-7.112, 40.0685) -> (-7.112, 184.3405)
  line L7 (-7.112, 184.3405) -> (42.418, 40.0685) construction
  line L8 (42.418, 184.3405) -> (-7.112, 40.0685) construction
  point P0 (17.653, 266.4975)
  point P1 (17.653, 112.2045)
  dimension "d174" = 49.53
  dimension "d175" = 144.272
  constraints: 14 end point, 5 midpoint, 2 parallel, 1 horizontal, 1 perpendicular
  measures "d174" distance of L3.start L3.end
  measures "d175" distance of L5.end L3.start
extrude "Extrusion27" cut sketch "Sketch28" against normal blind 19.05
sketch "Sketch29" plane through (-51.054, 22.1966, -108.7635) normal (0, 1, 0) x (1, 0, 0)
  line L0 (76.0783, 0) -> (26.0297, 0) projected
  line L1 (0, 110.998) -> (102.108, 110.998) projected
  line L2 (51.054, 110.998) -> (51.054, 0) construction
  line L3 (15.24, 105.791) -> (86.868, 105.791)
  line L4 (86.868, 105.791) -> (86.868, 5.207)
  line L5 (86.868, 5.207) -> (15.24, 5.207)
  line L6 (15.24, 5.207) -> (15.24, 105.791)
  line L7 (15.24, 105.791) -> (86.868, 5.207) construction
  line L8 (86.868, 105.791) -> (15.24, 5.207) construction
  point P0 (51.054, -108.7635)
  point P1 (51.054, 55.499)
  dimension "d178" = 71.628
  dimension "d179" = 100.584
  constraints: 14 end point, 5 midpoint, 2 parallel, 1 horizontal, 1 perpendicular
  measures "d178" distance of L3.start L3.end
  measures "d179" distance of L3.end L4.end
extrude "Extrusion28" cut sketch "Sketch29" against normal blind 25.4
body "Solid1"
